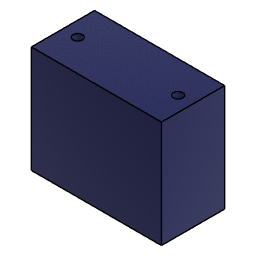
Sensor v2 (Autodesk Fusion 360 design; units mm, degrees)
Autodesk Fusion 360 part; units mm, degrees
sketch "Skizze1" plane through (0, 0, 0) normal (0, 0, 1) x (1, 0, 0)
  line L0 (0, 0) -> (-28, 0)
  line L1 (-28, 0) -> (-28, 13.6)
  line L2 (-28, 13.6) -> (0, 13.6)
  line L3 (0, 13.6) -> (0, 0)
  line L4 (-28, 6.8) -> (0, 6.8) construction
  circle A0 centre (-24.8, 6.8) radius 1
  circle A1 centre (-3.2, 6.8) radius 1
  line L5 (-14, 13.6) -> (-14, 0) construction
  dimension "d1" = 13.6
  dimension "d2" = 28
  dimension "d5" = 2
  dimension "d6" = 2
  dimension "d7" = 21.6
  constraint horizontal L0
  constraint vertical L1
  constraint horizontal L2
  constraint vertical L3
  constraint coincident L0.start L3.end
  constraint midpoint L1 L4.start
  constraint midpoint L3 L4.end
  constraint coincident L4 A0.centre
  constraint coincident L4 A1.centre
  constraint midpoint L2 L5.start
  constraint midpoint L0 L5.end
  constraint symmetric A0.centre A1.centre L5
  measures "d1" distance of L0.start L2.end
  measures "d2" distance of L0.start L0.end
  measures "d5" diameter of A0
  measures "d6" diameter of A1
  measures "d7" distance of A0.centre A1.centre
extrude "Extrusion1" add sketch "Skizze1" along normal blind 23 contours L0 L1 L2 L3 | A0 | A1
extrude "Extrusion2" cut sketch "Skizze1" along normal up to surface (8 mm away) from surface at 15 contours A0 | A1
